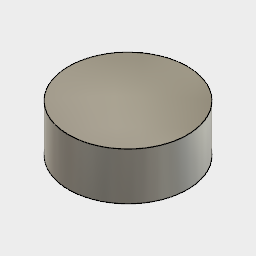
Disc Magnet (Autodesk Fusion 360 design; units mm, degrees)
Autodesk Fusion 360 part; units mm, degrees
sketch "Sketch1" plane through (0, 0, 0) normal (0, 1, 0) x (1, 0, 0)
  circle A0 centre (0, 0) radius 2.5
  dimension "d1" = 5
  measures "d1" diameter of A0
extrude "Extrude1" add sketch "Sketch1" along normal blind 2
